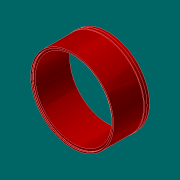
# Autodesk Inventor part: A1-19027-400-08 HCWI liner - pup
Saved by Autodesk Inventor 2017.3 (Build 213257000, 257)
## iProperties
Created: 2019-11-25
Part Number: A1-19027-400-08 HCWI liner - pup
Material: Iron, HCWI
Description: 28 1/2" ID x 1 1/4" WALL x 13 11/32" HCWI LINER PUP, ASTM A532 CLASS III TYPE A, PF#(TBD)
Document SubType Name: Modeling
Designer: GVD
Density: 7.33517 g/cm^3
Appearance: Iron Gray(1)
Mass: 184559 g
Surface Area: 17692.6 cm^2
Volume: 25160.8 cm^3
Author: GVD
Autodesk Inventor part; units mm, degrees
ref_plane "YZ Plane" through (0, 0, 0) normal (1, 0, 0) x (0, 1, 0)
ref_plane "XZ Plane" through (0, 0, 0) normal (0, 1, 0) x (-1, 0, 0)
ref_plane "XY Plane" through (0, 0, 0) normal (0, 0, 1) x (1, 0, 0)
sketch "Sketch1" plane through (0, 0, 0) normal (0, 0, 1) x (1, 0, 0)
  circle A0 centre (0, 0) radius 361.95
  circle A1 centre (0, 0) radius 393.7
  dimension "d0" = 723.9
  dimension "d1" = 787.4
  constraints: 2 centre point, 2 coincident
  measures "d0" diameter of A0
  measures "d1" diameter of A1
extrude "Extrusion1" add sketch "Sketch1" along normal blind 326
sketch "Sketch2" plane through (0, 0, 0) normal (0, 0, -1) x (-1, 0, 0)
  circle A0 centre (0, 0) radius 396.875
  circle A1 centre (0, 0) radius 393.7 projected
  dimension "d4" = 793.75
  constraints: 1 centre point, 1 coincident
  measures "d4" diameter of A0
extrude "Extrusion2" add sketch "Sketch2" against normal blind 50.8
sketch "Sketch3" plane through (0, 0, 0) normal (0, 0, -1) x (-1, 0, 0)
  circle A0 centre (0, 0) radius 396.875 projected
  circle A1 centre (0, 0) radius 393.446
  dimension "d7" = 786.892
  constraints: 1 centre point, 1 coincident
  measures "d7" diameter of A1
extrude "Extrusion3" cut sketch "Sketch3" against normal blind 25.4
chamfer "Chamfer1" distance 3.175 angle 45 1 edges at (-393.7, 0, 50.8)
sketch "Sketch4" plane through (0, 0, 326) normal (0, 0, 1) x (1, 0, 0)
  circle A0 centre (0, 0) radius 381
  circle A1 centre (0, 0) radius 393.7 projected
  dimension "d13" = 762
  constraints: 1 centre point, 1 coincident
  measures "d13" diameter of A0
extrude "Extrusion4" add sketch "Sketch4" along normal blind 12.7
fillet "Fillet1" radius 0.7937 2 edges at (-381, 0, 326) (393.446, 0, 25.4)
chamfer "Chamfer2" distance 0.7937 angle 45 1 edges at (-381, 0, 338.7)
equation "\"d10\" = -0.5 * d1 + 0.5 * d4"
body "Solid1"
